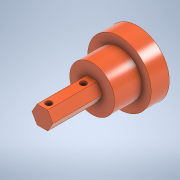
# Autodesk Inventor part: hexBushingForConnectorPiece
Saved by Autodesk Inventor 2022.2 (Build 262287000, 287)
## iProperties
Created: 2020-11-16
Part Number: hexBushingForConnectorPiece
Material: PC/ABS Plastic
Document SubType Name: Modeling
Designer: robst
Density: 0.357273 g/cm^3
Appearance: Smooth - Light Orange
Author: robst
Autodesk Inventor part; units mm, degrees
ref_plane "YZ Plane" through (0, 0, 0) normal (1, 0, 0) x (0, 1, 0)
ref_plane "XZ Plane" through (0, 0, 0) normal (0, 1, 0) x (-1, 0, 0)
ref_plane "XY Plane" through (0, 0, 0) normal (0, 0, 1) x (1, 0, 0)
sketch "Sketch1" plane through (0, 0, 0) normal (0, 0, 1) x (1, 0, 0)
  line L0 (7.3323, 0) -> (3.6662, -6.35)
  line L1 (3.6662, -6.35) -> (-3.6662, -6.35)
  line L2 (-3.6662, -6.35) -> (-7.3323, 0)
  line L3 (-7.3323, 0) -> (-3.6662, 6.35)
  line L4 (-3.6662, 6.35) -> (3.6662, 6.35)
  line L5 (3.6662, 6.35) -> (7.3323, 0)
  point P0 (0, 0)
  point P1 (0, 0)
  dimension "d0" = 12.7
  constraints: 12 end point, 1 coincident, 1 horizontal, 13 other
  measures "d0" distance between parallel lines of L1 L4
extrude "Extrusion1" add sketch "Sketch1" along normal mid plane 34.925
sketch "Sketch2" plane through (0, 0, -17.4625) normal (0, 0, -1) x (-1, 0, 0)
  circle A0 centre (0, 0) radius 15.748
  dimension "d3" = 31.496
  constraints: 1 centre point, 1 coincident
  measures "d3" diameter of A0
extrude "Extrusion2" add sketch "Sketch2" along normal blind 19.05
sketch "Sketch3" plane through (0, 0, -36.5125) normal (0, 0, -1) x (-1, 0, 0)
  circle A0 centre (0, 0) radius 22.225
  dimension "d6" = 44.45
  constraints: 1 centre point, 1 coincident
  measures "d6" diameter of A0
extrude "Extrusion3" add sketch "Sketch3" along normal blind 12.7
sketch "Sketch4" plane through (0, 0, -49.2125) normal (0, 0, -1) x (-1, 0, 0)
  circle A0 centre (0, 0) radius 16.51 construction
  line L0 (-13.6277, 3.4249) -> (-13.7163, 2.7889)
  line L1 (-13.7163, 2.7889) -> (-15.8691, 3.0889)
  spline S0 degree 2 poles (-15.8691, 3.0889) (-16.1301, 3.1253) (-16.5854, 3.1389) (-16.7302, 3.0842) knots 0 0 0 1 2 2 2
  spline S1 degree 2 poles (-16.7302, 3.0842) (-16.8837, 3.0267) (-17.061, 2.7687) (-17.0939, 2.5323) knots 0 0 0 1 2 2 2
  spline S2 degree 2 poles (-17.0939, 2.5323) (-17.1269, 2.2958) (-16.944, 1.759) (-16.7737, 1.4901) knots 0 0 0 1 2 2 2
  line L2 (-16.7737, 1.4901) -> (-13.9522, 1.0968)
  line L3 (-13.9522, 1.0968) -> (-14.0408, 0.4607)
  line L4 (-14.0408, 0.4607) -> (-19.2964, 1.1933)
  line L5 (-19.2964, 1.1933) -> (-19.2078, 1.8293)
  line L6 (-19.2078, 1.8293) -> (-17.3078, 1.5645)
  spline S3 degree 2 poles (-17.3078, 1.5645) (-17.5249, 1.8857) (-17.7172, 2.4737) (-17.6741, 2.7835) knots 0 0 0 1 2 2 2
  spline S4 degree 2 poles (-17.6741, 2.7835) (-17.5968, 3.338) (-16.7753, 3.8636) (-16.0781, 3.7665) knots 0 0 0 1 2 2 2
  line L7 (-16.0781, 3.7665) -> (-13.6277, 3.4249)
  spline S5 degree 2 poles (-12.6332, 5.765) (-12.9956, 4.9261) (-14.335, 4.4105) (-15.2042, 4.786) knots 0 0 0 1 2 2 2
  spline S6 degree 2 poles (-15.2042, 4.786) (-16.0582, 5.155) (-16.6841, 6.4882) (-16.3723, 7.21) knots 0 0 0 1 2 2 2
  spline S7 degree 2 poles (-16.3723, 7.21) (-16.2318, 7.535) (-15.8257, 7.956) (-15.5455, 8.0547) knots 0 0 0 1 2 2 2
  spline S8 degree 2 poles (-15.5455, 8.0547) (-15.2635, 8.1571) (-14.5988, 8.1076) (-14.1793, 7.9264) knots 0 0 0 1 2 2 2
  line L8 (-14.1793, 7.9264) -> (-13.8581, 7.7876)
  line L9 (-13.8581, 7.7876) -> (-14.9046, 5.3652)
  spline S9 degree 2 poles (-14.9046, 5.3652) (-14.2962, 5.1023) (-13.3855, 5.4353) (-13.1504, 5.9795) knots 0 0 0 1 2 2 2
  spline S10 degree 2 poles (-13.1504, 5.9795) (-13.0671, 6.1723) (-12.9924, 6.5839) (-12.9951, 6.7645) knots 0 0 0 1 2 2 2
  spline S11 degree 2 poles (-12.9951, 6.7645) (-13.0021, 6.9559) (-13.0397, 7.2322) (-13.0691, 7.3301) knots 0 0 0 1 2 2 2
  line L10 (-13.0691, 7.3301) -> (-13.0545, 7.3641)
  line L11 (-13.0545, 7.3641) -> (-12.412, 7.0866)
  spline S12 degree 2 poles (-12.412, 7.0866) (-12.4145, 6.9666) (-12.4275, 6.6045) (-12.4457, 6.4688) knots 0 0 0 1 2 2 2
  spline S13 degree 2 poles (-12.4457, 6.4688) (-12.47, 6.2776) (-12.5417, 5.9767) (-12.6332, 5.765) knots 0 0 0 1 2 2 2
  spline S14 degree 2 poles (-14.556, 7.4074) (-14.7973, 7.5027) (-15.1874, 7.5547) (-15.3454, 7.5108) knots 0 0 0 1 2 2 2
  spline S15 degree 2 poles (-15.3454, 7.5108) (-15.5218, 7.4659) (-15.8004, 7.2051) (-15.9032, 6.967) knots 0 0 0 1 2 2 2
  spline S16 degree 2 poles (-15.9032, 6.967) (-16.0045, 6.7327) (-16.0067, 6.3435) (-15.9294, 6.1487) knots 0 0 0 1 2 2 2
  spline S17 degree 2 poles (-15.9294, 6.1487) (-15.8467, 5.956) (-15.5692, 5.6747) (-15.3543, 5.5595) knots 0 0 0 1 2 2 2
  line L12 (-15.3543, 5.5595) -> (-14.556, 7.4074)
  line L13 (-9.9787, 9.9228) -> (-10.4619, 9.3025)
  line L14 (-10.4619, 9.3025) -> (-12.1613, 9.4521)
  line L15 (-12.1613, 9.4521) -> (-11.6155, 7.8216)
  line L16 (-11.6155, 7.8216) -> (-12.0633, 7.2467)
  line L17 (-12.0633, 7.2467) -> (-12.7419, 9.4504)
  line L18 (-12.7419, 9.4504) -> (-15.063, 9.599)
  line L19 (-15.063, 9.599) -> (-14.5799, 10.2193)
  line L20 (-14.5799, 10.2193) -> (-12.8927, 10.0741)
  line L21 (-12.8927, 10.0741) -> (-13.4339, 11.6905)
  line L22 (-13.4339, 11.6905) -> (-12.9861, 12.2654)
  line L23 (-12.9861, 12.2654) -> (-12.3089, 10.0733)
  line L24 (-12.3089, 10.0733) -> (-9.9787, 9.9228)
  spline S18 degree 2 poles (-7.7436, 13.5957) (-7.5175, 13.2918) (-7.4023, 12.6541) (-7.4808, 12.3596) knots 0 0 0 1 2 2 2
  spline S19 degree 2 poles (-7.4808, 12.3596) (-7.5794, 12.0093) (-7.9915, 11.4666) (-8.4077, 11.157) knots 0 0 0 1 2 2 2
  line L25 (-8.4077, 11.157) -> (-9.5769, 10.2872)
  line L26 (-9.5769, 10.2872) -> (-12.609, 14.3631)
  line L27 (-12.609, 14.3631) -> (-11.529, 15.1666)
  spline S20 degree 2 poles (-11.529, 15.1666) (-11.093, 15.4909) (-10.6152, 15.7591) (-10.336, 15.7975) knots 0 0 0 1 2 2 2
  spline S21 degree 2 poles (-10.336, 15.7975) (-10.0287, 15.8465) (-9.5446, 15.6166) (-9.3529, 15.359) knots 0 0 0 1 2 2 2
  spline S22 degree 2 poles (-9.3529, 15.359) (-9.1392, 15.0716) (-9.104, 14.3897) (-9.2757, 14.0619) knots 0 0 0 1 2 2 2
  line L28 (-9.2757, 14.0619) -> (-9.2609, 14.0421)
  spline S23 degree 2 poles (-9.2609, 14.0421) (-8.8239, 14.2133) (-8.0335, 13.9854) (-7.7436, 13.5957) knots 0 0 0 1 2 2 2
  spline S24 degree 2 poles (-8.2912, 13.1524) (-8.4632, 13.3836) (-8.8165, 13.5826) (-9.0933, 13.5408) knots 0 0 0 1 2 2 2
  spline S25 degree 2 poles (-9.0933, 13.5408) (-9.2712, 13.5111) (-9.6046, 13.3246) (-9.8853, 13.1158) knots 0 0 0 1 2 2 2
  line L29 (-9.8853, 13.1158) -> (-10.4997, 12.6587)
  line L30 (-10.4997, 12.6587) -> (-9.3792, 11.1526)
  line L31 (-9.3792, 11.1526) -> (-8.9399, 11.4794)
  spline S26 degree 2 poles (-8.9399, 11.4794) (-8.5832, 11.7448) (-8.2228, 12.1155) (-8.1429, 12.3391) knots 0 0 0 1 2 2 2
  spline S27 degree 2 poles (-8.1429, 12.3391) (-8.072, 12.5612) (-8.1315, 12.9377) (-8.2912, 13.1524) knots 0 0 0 1 2 2 2
  spline S28 degree 2 poles (-9.8612, 14.8628) (-9.9693, 15.0081) (-10.2306, 15.1524) (-10.3863, 15.1341) knots 0 0 0 1 2 2 2
  spline S29 degree 2 poles (-10.3863, 15.1341) (-10.5725, 15.1085) (-10.9174, 14.9032) (-11.2048, 14.6894) knots 0 0 0 1 2 2 2
  line L32 (-11.2048, 14.6894) -> (-11.7234, 14.3036)
  line L33 (-11.7234, 14.3036) -> (-10.8363, 13.1113)
  line L34 (-10.8363, 13.1113) -> (-10.222, 13.5683)
  spline S30 degree 2 poles (-10.222, 13.5683) (-9.9676, 13.7575) (-9.7658, 13.9897) (-9.6985, 14.1681) knots 0 0 0 1 2 2 2
  spline S31 degree 2 poles (-9.6985, 14.1681) (-9.6319, 14.3407) (-9.7187, 14.6712) (-9.8612, 14.8628) knots 0 0 0 1 2 2 2
  line L35 (-3.4638, 13.6147) -> (-4.066, 13.3916)
  line L36 (-4.066, 13.3916) -> (-4.2118, 13.7853)
  spline S32 degree 2 poles (-4.2118, 13.7853) (-4.3997, 13.4391) (-4.8047, 13.0037) (-5.1135, 12.8893) knots 0 0 0 1 2 2 2
  spline S33 degree 2 poles (-5.1135, 12.8893) (-5.3451, 12.8035) (-5.8154, 12.8049) (-6.0274, 12.9151) knots 0 0 0 1 2 2 2
  spline S34 degree 2 poles (-6.0274, 12.9151) (-6.2433, 13.0239) (-6.6006, 13.4666) (-6.735, 13.8295) knots 0 0 0 1 2 2 2
  line L37 (-6.735, 13.8295) -> (-7.5946, 16.1495)
  line L38 (-7.5946, 16.1495) -> (-6.9924, 16.3726)
  line L39 (-6.9924, 16.3726) -> (-6.2372, 14.3344)
  spline S35 degree 2 poles (-6.2372, 14.3344) (-6.1314, 14.0488) (-5.9502, 13.69) (-5.8253, 13.5782) knots 0 0 0 1 2 2 2
  spline S36 degree 2 poles (-5.8253, 13.5782) (-5.7005, 13.4665) (-5.4024, 13.432) (-5.1669, 13.5193) knots 0 0 0 1 2 2 2
  spline S37 degree 2 poles (-5.1669, 13.5193) (-4.9469, 13.6008) (-4.5419, 14.0362) (-4.4006, 14.2949) knots 0 0 0 1 2 2 2
  line L40 (-4.4006, 14.2949) -> (-5.3903, 16.9662)
  line L41 (-5.3903, 16.9662) -> (-4.7881, 17.1893)
  line L42 (-4.7881, 17.1893) -> (-3.4638, 13.6147)
  spline S38 degree 2 poles (-1.5215, 13.7959) (-1.9023, 13.7557) (-2.583, 13.8908) (-2.8121, 13.9825) knots 0 0 0 1 2 2 2
  line L43 (-2.8121, 13.9825) -> (-2.8878, 14.6989)
  line L44 (-2.8878, 14.6989) -> (-2.855, 14.7024)
  spline S39 degree 2 poles (-2.855, 14.7024) (-2.7662, 14.6455) (-2.5287, 14.5133) (-2.3354, 14.4468) knots 0 0 0 1 2 2 2
  spline S40 degree 2 poles (-2.3354, 14.4468) (-2.1676, 14.3859) (-1.7624, 14.3128) (-1.5536, 14.3348) knots 0 0 0 1 2 2 2
  spline S41 degree 2 poles (-1.5536, 14.3348) (-1.4022, 14.3508) (-1.0615, 14.4572) (-0.9857, 14.5231) knots 0 0 0 1 2 2 2
  spline S42 degree 2 poles (-0.9857, 14.5231) (-0.8752, 14.6135) (-0.7874, 14.8008) (-0.8064, 14.9809) knots 0 0 0 1 2 2 2
  spline S43 degree 2 poles (-0.8064, 14.9809) (-0.8302, 15.2061) (-1.1005, 15.4135) (-1.4239, 15.4579) knots 0 0 0 1 2 2 2
  spline S44 degree 2 poles (-1.4239, 15.4579) (-1.5498, 15.4736) (-1.9514, 15.514) (-2.124, 15.5413) knots 0 0 0 1 2 2 2
  spline S45 degree 2 poles (-2.124, 15.5413) (-2.5714, 15.6224) (-3.0198, 16.1049) (-3.0591, 16.4774) knots 0 0 0 1 2 2 2
  spline S46 degree 2 poles (-3.0591, 16.4774) (-3.1136, 16.9932) (-2.4078, 17.7177) (-1.7691, 17.7852) knots 0 0 0 1 2 2 2
  spline S47 degree 2 poles (-1.7691, 17.7852) (-1.4539, 17.8185) (-0.7988, 17.7304) (-0.5693, 17.6346) knots 0 0 0 1 2 2 2
  line L45 (-0.5693, 17.6346) -> (-0.497, 16.9509)
  line L46 (-0.497, 16.9509) -> (-0.5298, 16.9474)
  spline S48 degree 2 poles (-0.5298, 16.9474) (-0.7962, 17.118) (-1.4177, 17.28) (-1.7247, 17.2476) knots 0 0 0 1 2 2 2
  spline S49 degree 2 poles (-1.7247, 17.2476) (-2.04, 17.2143) (-2.4458, 16.9023) (-2.4177, 16.6362) knots 0 0 0 1 2 2 2
  spline S50 degree 2 poles (-2.4177, 16.6362) (-2.3922, 16.3947) (-2.1096, 16.1886) (-1.8153, 16.1452) knots 0 0 0 1 2 2 2
  spline S51 degree 2 poles (-1.8153, 16.1452) (-1.6722, 16.123) (-1.3123, 16.0865) (-1.1151, 16.0618) knots 0 0 0 1 2 2 2
  spline S52 degree 2 poles (-1.1151, 16.0618) (-0.6863, 15.9995) (-0.2091, 15.5573) (-0.1645, 15.1356) knots 0 0 0 1 2 2 2
  spline S53 degree 2 poles (-0.1645, 15.1356) (-0.1386, 14.89) (-0.2852, 14.4357) (-0.4566, 14.2562) knots 0 0 0 1 2 2 2
  spline S54 degree 2 poles (-0.4566, 14.2562) (-0.6395, 14.0671) (-1.1326, 13.837) (-1.5215, 13.7959) knots 0 0 0 1 2 2 2
  line L47 (3.5043, 13.6075) -> (2.8688, 13.6998)
  line L48 (2.8688, 13.6998) -> (3.1814, 15.8509)
  spline S55 degree 2 poles (3.1814, 15.8509) (3.2193, 16.1116) (3.2355, 16.5668) (3.1817, 16.7119) knots 0 0 0 1 2 2 2
  spline S56 degree 2 poles (3.1817, 16.7119) (3.125, 16.8658) (2.8681, 17.0445) (2.6319, 17.0789) knots 0 0 0 1 2 2 2
  spline S57 degree 2 poles (2.6319, 17.0789) (2.3956, 17.1132) (1.8578, 16.9334) (1.5878, 16.7647) knots 0 0 0 1 2 2 2
  line L49 (1.5878, 16.7647) -> (1.1781, 13.9455)
  line L50 (1.1781, 13.9455) -> (0.5426, 14.0379)
  line L51 (0.5426, 14.0379) -> (1.3057, 19.2892)
  line L52 (1.3057, 19.2892) -> (1.9413, 19.1968)
  line L53 (1.9413, 19.1968) -> (1.6654, 17.2984)
  spline S58 degree 2 poles (1.6654, 17.2984) (1.9878, 17.5136) (2.5769, 17.7025) (2.8865, 17.6575) knots 0 0 0 1 2 2 2
  spline S59 degree 2 poles (2.8865, 17.6575) (3.4406, 17.577) (3.9614, 16.7525) (3.8601, 16.0559) knots 0 0 0 1 2 2 2
  line L54 (3.8601, 16.0559) -> (3.5043, 13.6075)
  line L55 (4.9605, 13.0636) -> (4.355, 13.2777)
  line L56 (4.355, 13.2777) -> (5.626, 16.8717)
  line L57 (5.626, 16.8717) -> (6.2315, 16.6575)
  line L58 (6.2315, 16.6575) -> (4.9605, 13.0636)
  line L59 (6.4855, 17.2401) -> (5.7986, 17.4831)
  line L60 (5.7986, 17.4831) -> (6.0209, 18.1118)
  line L61 (6.0209, 18.1118) -> (6.7079, 17.8689)
  line L62 (6.7079, 17.8689) -> (6.4855, 17.2401)
  line L63 (8.428, 11.2433) -> (7.8757, 11.571)
  line L64 (7.8757, 11.571) -> (8.9849, 13.4403)
  spline S60 degree 2 poles (8.9849, 13.4403) (9.1193, 13.6669) (9.3079, 14.0816) (9.3135, 14.2362) knots 0 0 0 1 2 2 2
  spline S61 degree 2 poles (9.3135, 14.2362) (9.3198, 14.4001) (9.1504, 14.6633) (8.9451, 14.7851) knots 0 0 0 1 2 2 2
  spline S62 degree 2 poles (8.9451, 14.7851) (8.7398, 14.907) (8.174, 14.9458) (7.8601, 14.8928) knots 0 0 0 1 2 2 2
  line L65 (7.8601, 14.8928) -> (6.4064, 12.4428)
  line L66 (6.4064, 12.4428) -> (5.8542, 12.7705)
  line L67 (5.8542, 12.7705) -> (7.7994, 16.0489)
  line L68 (7.7994, 16.0489) -> (8.3517, 15.7212)
  line L69 (8.3517, 15.7212) -> (8.1353, 15.3565)
  spline S63 degree 2 poles (8.1353, 15.3565) (8.5155, 15.4325) (9.1321, 15.3826) (9.4012, 15.223) knots 0 0 0 1 2 2 2
  spline S64 degree 2 poles (9.4012, 15.223) (9.8826, 14.9373) (10.0497, 13.9765) (9.6905, 13.3711) knots 0 0 0 1 2 2 2
  line L70 (9.6905, 13.3711) -> (8.428, 11.2433)
  spline S65 degree 2 poles (8.7739, 10.1635) (8.7983, 10.0959) (8.9055, 9.8514) (8.9892, 9.7095) knots 0 0 0 1 2 2 2
  spline S66 degree 2 poles (8.9892, 9.7095) (9.0782, 9.5499) (9.2463, 9.2951) (9.3682, 9.1668) knots 0 0 0 1 2 2 2
  spline S67 degree 2 poles (9.3682, 9.1668) (9.5723, 8.9518) (9.9692, 8.761) (10.1501, 8.7737) knots 0 0 0 1 2 2 2
  spline S68 degree 2 poles (10.1501, 8.7737) (10.3281, 8.7895) (10.6533, 8.9791) (10.8235, 9.1406) knots 0 0 0 1 2 2 2
  line L71 (10.8235, 9.1406) -> (11.0653, 9.3702)
  spline S69 degree 2 poles (11.0653, 9.3702) (10.7226, 9.4024) (10.2243, 9.6163) (9.9664, 9.8879) knots 0 0 0 1 2 2 2
  spline S70 degree 2 poles (9.9664, 9.8879) (9.5186, 10.3597) (9.6901, 11.584) (10.3499, 12.2104) knots 0 0 0 1 2 2 2
  spline S71 degree 2 poles (10.3499, 12.2104) (10.6932, 12.5364) (11.4089, 12.8469) (11.75, 12.8642) knots 0 0 0 1 2 2 2
  spline S72 degree 2 poles (11.75, 12.8642) (12.0736, 12.8762) (12.673, 12.6335) (12.8884, 12.4066) knots 0 0 0 1 2 2 2
  spline S73 degree 2 poles (12.8884, 12.4066) (13.0925, 12.1917) (13.2886, 11.7818) (13.3462, 11.5357) knots 0 0 0 1 2 2 2
  line L72 (13.3462, 11.5357) -> (13.4882, 11.6194)
  line L73 (13.4882, 11.6194) -> (13.9048, 11.1806)
  line L74 (13.9048, 11.1806) -> (11.4568, 8.8563)
  spline S74 degree 2 poles (11.4568, 8.8563) (10.7522, 8.1874) (9.5143, 8.1758) (8.9162, 8.8058) knots 0 0 0 1 2 2 2
  spline S75 degree 2 poles (8.9162, 8.8058) (8.7235, 9.0088) (8.3867, 9.4951) (8.2675, 9.7282) knots 0 0 0 1 2 2 2
  line L75 (8.2675, 9.7282) -> (8.7512, 10.1874)
  line L76 (8.7512, 10.1874) -> (8.7739, 10.1635)
  line L77 (11.4475, 9.733) -> (12.9671, 11.1758)
  spline S76 degree 2 poles (12.9671, 11.1758) (12.8863, 11.4283) (12.6802, 11.7889) (12.5413, 11.9352) knots 0 0 0 1 2 2 2
  spline S77 degree 2 poles (12.5413, 11.9352) (12.2068, 12.2875) (11.3018, 12.2003) (10.8152, 11.7383) knots 0 0 0 1 2 2 2
  spline S78 degree 2 poles (10.8152, 11.7383) (10.3554, 11.3018) (10.1667, 10.5379) (10.4955, 10.1916) knots 0 0 0 1 2 2 2
  spline S79 degree 2 poles (10.4955, 10.1916) (10.6684, 10.0095) (11.1745, 9.7634) (11.4475, 9.733) knots 0 0 0 1 2 2 2
  line L78 (17.0752, 7.1971) -> (15.958, 9.2793)
  line L79 (15.958, 9.2793) -> (14.6956, 8.602)
  line L80 (14.6956, 8.602) -> (15.7661, 6.6068)
  line L81 (15.7661, 6.6068) -> (15.2365, 6.3227)
  line L82 (15.2365, 6.3227) -> (14.166, 8.3178)
  line L83 (14.166, 8.3178) -> (12.0113, 7.1617)
  line L84 (12.0113, 7.1617) -> (11.6921, 7.7566)
  line L85 (11.6921, 7.7566) -> (16.1684, 10.1584)
  line L86 (16.1684, 10.1584) -> (17.6048, 7.4812)
  line L87 (17.6048, 7.4812) -> (17.0752, 7.1971)
  spline S80 degree 2 poles (15.8501, 1.9288) (14.9117, 1.7112) (13.6798, 2.3763) (13.5049, 3.1302) knots 0 0 0 1 2 2 2
  spline S81 degree 2 poles (13.5049, 3.1302) (13.3254, 3.9042) (14.1746, 5.0351) (15.0809, 5.2453) knots 0 0 0 1 2 2 2
  spline S82 degree 2 poles (15.0809, 5.2453) (16.0112, 5.4611) (17.2539, 4.7858) (17.427, 4.0399) knots 0 0 0 1 2 2 2
  spline S83 degree 2 poles (17.427, 4.0399) (17.6018, 3.286) (16.7845, 2.1456) (15.8501, 1.9288) knots 0 0 0 1 2 2 2
  spline S84 degree 2 poles (15.7003, 2.5745) (16.4222, 2.7419) (17.0021, 3.43) (16.8896, 3.9153) knots 0 0 0 1 2 2 2
  spline S85 degree 2 poles (16.8896, 3.9153) (16.777, 4.4005) (15.9525, 4.7671) (15.2306, 4.5997) knots 0 0 0 1 2 2 2
  spline S86 degree 2 poles (15.2306, 4.5997) (14.5288, 4.4369) (13.9298, 3.7401) (14.0423, 3.2549) knots 0 0 0 1 2 2 2
  spline S87 degree 2 poles (14.0423, 3.2549) (14.1539, 2.7736) (14.9865, 2.4089) (15.7003, 2.5745) knots 0 0 0 1 2 2 2
  line L88 (17.0983, -1.1737) -> (17.0982, -1.1408)
  spline S88 degree 2 poles (17.0982, -1.1408) (17.1185, -1.0666) (17.1263, -0.906) (17.1259, -0.7949) knots 0 0 0 1 2 2 2
  spline S89 degree 2 poles (17.1259, -0.7949) (17.1251, -0.5355) (16.8971, -0.0258) (16.6741, 0.2041) knots 0 0 0 1 2 2 2
  line L89 (16.6741, 0.2041) -> (13.9695, 0.1957)
  line L90 (13.9695, 0.1957) -> (13.9675, 0.8379)
  line L91 (13.9675, 0.8379) -> (17.7795, 0.8497)
  line L92 (17.7795, 0.8497) -> (17.7815, 0.2075)
  line L93 (17.7815, 0.2075) -> (17.2134, 0.2058)
  spline S90 degree 2 poles (17.2134, 0.2058) (17.5274, -0.1432) (17.7842, -0.6652) (17.785, -0.9122) knots 0 0 0 1 2 2 2
  spline S91 degree 2 poles (17.785, -0.9122) (17.7853, -1.011) (17.7774, -1.1098) (17.7652, -1.1716) knots 0 0 0 1 2 2 2
  line L94 (17.7652, -1.1716) -> (17.0983, -1.1737)
  spline S92 degree 2 poles (13.4014, -3.6335) (13.5168, -3.1532) (14.0363, -2.4185) (14.4317, -2.2002) knots 0 0 0 1 2 2 2
  spline S93 degree 2 poles (14.4317, -2.2002) (14.8231, -1.981) (15.8617, -1.8876) (16.4861, -2.0377) knots 0 0 0 1 2 2 2
  spline S94 degree 2 poles (16.4861, -2.0377) (17.1066, -2.1868) (17.9512, -2.7243) (18.2193, -3.1062) knots 0 0 0 1 2 2 2
  spline S95 degree 2 poles (18.2193, -3.1062) (18.4803, -3.4823) (18.6342, -4.3745) (18.514, -4.8749) knots 0 0 0 1 2 2 2
  spline S96 degree 2 poles (18.514, -4.8749) (18.4544, -5.123) (18.2775, -5.542) (18.1772, -5.7127) knots 0 0 0 1 2 2 2
  spline S97 degree 2 poles (18.1772, -5.7127) (18.0867, -5.8603) (17.8587, -6.1569) (17.7312, -6.2999) knots 0 0 0 1 2 2 2
  line L95 (17.7312, -6.2999) -> (16.9387, -6.1094)
  line L96 (16.9387, -6.1094) -> (16.9512, -6.0574)
  spline S98 degree 2 poles (16.9512, -6.0574) (17.0524, -5.9885) (17.342, -5.7702) (17.4972, -5.6001) knots 0 0 0 1 2 2 2
  spline S99 degree 2 poles (17.4972, -5.6001) (17.6465, -5.4369) (17.8853, -5.0244) (17.9546, -4.7362) knots 0 0 0 1 2 2 2
  spline S100 degree 2 poles (17.9546, -4.7362) (18.0306, -4.42) (17.906, -3.7931) (17.7088, -3.5213) knots 0 0 0 1 2 2 2
  spline S101 degree 2 poles (17.7088, -3.5213) (17.5067, -3.2525) (16.798, -2.8366) (16.3216, -2.7222) knots 0 0 0 1 2 2 2
  spline S102 degree 2 poles (16.3216, -2.7222) (15.8133, -2.6) (15.0221, -2.6681) (14.719, -2.8197) knots 0 0 0 1 2 2 2
  spline S103 degree 2 poles (14.719, -2.8197) (14.4248, -2.9691) (14.0429, -3.4659) (13.9679, -3.7781) knots 0 0 0 1 2 2 2
  spline S104 degree 2 poles (13.9679, -3.7781) (13.8996, -4.0623) (13.9233, -4.5803) (13.9821, -4.7934) knots 0 0 0 1 2 2 2
  spline S105 degree 2 poles (13.9821, -4.7934) (14.0429, -4.9985) (14.1946, -5.3187) (14.2524, -5.413) knots 0 0 0 1 2 2 2
  line L97 (14.2524, -5.413) -> (14.2408, -5.461)
  line L98 (14.2408, -5.461) -> (13.4563, -5.2725)
  spline S106 degree 2 poles (13.4563, -5.2725) (13.4197, -5.0901) (13.3489, -4.7682) (13.3339, -4.5487) knots 0 0 0 1 2 2 2
  spline S107 degree 2 poles (13.3339, -4.5487) (13.3138, -4.3152) (13.3302, -3.9297) (13.4014, -3.6335) knots 0 0 0 1 2 2 2
  spline S108 degree 2 poles (12.934, -9.3626) (12.0979, -8.8841) (11.6468, -7.5588) (12.0312, -6.8871) knots 0 0 0 1 2 2 2
  spline S109 degree 2 poles (12.0312, -6.8871) (12.4258, -6.1975) (13.8174, -5.9456) (14.6249, -6.4076) knots 0 0 0 1 2 2 2
  spline S110 degree 2 poles (14.6249, -6.4076) (15.4539, -6.882) (15.906, -8.2221) (15.5257, -8.8867) knots 0 0 0 1 2 2 2
  spline S111 degree 2 poles (15.5257, -8.8867) (15.1413, -9.5584) (13.7665, -9.839) (12.934, -9.3626) knots 0 0 0 1 2 2 2
  spline S112 degree 2 poles (13.2632, -8.7873) (13.9063, -9.1553) (14.7995, -9.0451) (15.0469, -8.6127) knots 0 0 0 1 2 2 2
  spline S113 degree 2 poles (15.0469, -8.6127) (15.2943, -8.1804) (14.9389, -7.3509) (14.2957, -6.9829) knots 0 0 0 1 2 2 2
  spline S114 degree 2 poles (14.2957, -6.9829) (13.6704, -6.6251) (12.7574, -6.7287) (12.51, -7.161) knots 0 0 0 1 2 2 2
  spline S115 degree 2 poles (12.51, -7.161) (12.2646, -7.5898) (12.6272, -8.4234) (13.2632, -8.7873) knots 0 0 0 1 2 2 2
  line L99 (8.7251, -11.0143) -> (9.1827, -10.5637)
  line L100 (9.1827, -10.5637) -> (10.7078, -12.1125)
  spline S116 degree 2 poles (10.7078, -12.1125) (10.8927, -12.3003) (11.2456, -12.5883) (11.3937, -12.6331) knots 0 0 0 1 2 2 2
  spline S117 degree 2 poles (11.3937, -12.6331) (11.5505, -12.6809) (11.8482, -12.5842) (12.0183, -12.4167) knots 0 0 0 1 2 2 2
  spline S118 degree 2 poles (12.0183, -12.4167) (12.1885, -12.2492) (12.3702, -11.712) (12.3988, -11.3949) knots 0 0 0 1 2 2 2
  line L101 (12.3988, -11.3949) -> (10.4001, -9.3651)
  line L102 (10.4001, -9.3651) -> (10.8577, -8.9145)
  line L103 (10.8577, -8.9145) -> (13.5323, -11.6308)
  line L104 (13.5323, -11.6308) -> (13.0747, -12.0813)
  line L105 (13.0747, -12.0813) -> (12.7772, -11.7792)
  spline S119 degree 2 poles (12.7772, -11.7792) (12.7538, -12.1662) (12.5485, -12.7497) (12.3255, -12.9692) knots 0 0 0 1 2 2 2
  spline S120 degree 2 poles (12.3255, -12.9692) (11.9266, -13.3621) (10.955, -13.2789) (10.4611, -12.7773) knots 0 0 0 1 2 2 2
  line L106 (10.4611, -12.7773) -> (8.7251, -11.0143)
  line L107 (5.3806, -12.9805) -> (5.944, -12.6722)
  line L108 (5.944, -12.6722) -> (6.9874, -14.579)
  spline S121 degree 2 poles (6.9874, -14.579) (7.1139, -14.8101) (7.3746, -15.1836) (7.5048, -15.2673) knots 0 0 0 1 2 2 2
  spline S122 degree 2 poles (7.5048, -15.2673) (7.6426, -15.3561) (7.9554, -15.3445) (8.1648, -15.2299) knots 0 0 0 1 2 2 2
  spline S123 degree 2 poles (8.1648, -15.2299) (8.3743, -15.1153) (8.696, -14.6483) (8.8102, -14.3511) knots 0 0 0 1 2 2 2
  line L109 (8.8102, -14.3511) -> (7.4427, -11.8521)
  line L110 (7.4427, -11.8521) -> (8.0061, -11.5438)
  line L111 (8.0061, -11.5438) -> (9.836, -14.8879)
  line L112 (9.836, -14.8879) -> (9.2727, -15.1962)
  line L113 (9.2727, -15.1962) -> (9.0691, -14.8242)
  spline S124 degree 2 poles (9.0691, -14.8242) (8.9408, -15.1901) (8.5837, -15.6952) (8.3092, -15.8454) knots 0 0 0 1 2 2 2
  spline S125 degree 2 poles (8.3092, -15.8454) (7.8181, -16.1142) (6.9062, -15.7684) (6.5683, -15.1509) knots 0 0 0 1 2 2 2
  line L114 (6.5683, -15.1509) -> (5.3806, -12.9805)
  spline S126 degree 2 poles (2.9092, -13.5782) (3.7988, -13.3687) (5.0115, -14.1361) (5.2287, -15.0577) knots 0 0 0 1 2 2 2
  spline S127 degree 2 poles (5.2287, -15.0577) (5.442, -15.9633) (4.7454, -17.2609) (3.98, -17.4412) knots 0 0 0 1 2 2 2
  spline S128 degree 2 poles (3.98, -17.4412) (3.6354, -17.5224) (3.0553, -17.4476) (2.8089, -17.2815) knots 0 0 0 1 2 2 2
  spline S129 degree 2 poles (2.8089, -17.2815) (2.5585, -17.1163) (2.2017, -16.5533) (2.0969, -16.1085) knots 0 0 0 1 2 2 2
  line L115 (2.0969, -16.1085) -> (2.0167, -15.7679)
  line L116 (2.0167, -15.7679) -> (4.5852, -15.1628)
  spline S130 degree 2 poles (4.5852, -15.1628) (4.4332, -14.5176) (3.6226, -13.9854) (3.0456, -14.1213) knots 0 0 0 1 2 2 2
  spline S131 degree 2 poles (3.0456, -14.1213) (2.8413, -14.1695) (2.4663, -14.3551) (2.323, -14.465) knots 0 0 0 1 2 2 2
  spline S132 degree 2 poles (2.323, -14.465) (2.1736, -14.5848) (1.9742, -14.7797) (1.9132, -14.8618) knots 0 0 0 1 2 2 2
  line L117 (1.9132, -14.8618) -> (1.8771, -14.8703)
  line L118 (1.8771, -14.8703) -> (1.7167, -14.1891)
  spline S133 degree 2 poles (1.7167, -14.1891) (1.8145, -14.1195) (2.1128, -13.9139) (2.2325, -13.8476) knots 0 0 0 1 2 2 2
  spline S134 degree 2 poles (2.2325, -13.8476) (2.4006, -13.7531) (2.6848, -13.6311) (2.9092, -13.5782) knots 0 0 0 1 2 2 2
  spline S135 degree 2 poles (2.7381, -16.1012) (2.8056, -16.3518) (2.9966, -16.6959) (3.1261, -16.7965) knots 0 0 0 1 2 2 2
  spline S136 degree 2 poles (3.1261, -16.7965) (3.2673, -16.9112) (3.6428, -16.9793) (3.8953, -16.9198) knots 0 0 0 1 2 2 2
  spline S137 degree 2 poles (3.8953, -16.9198) (4.1437, -16.8613) (4.4574, -16.6309) (4.5676, -16.4526) knots 0 0 0 1 2 2 2
  spline S138 degree 2 poles (4.5676, -16.4526) (4.673, -16.2713) (4.7332, -15.8807) (4.6975, -15.6396) knots 0 0 0 1 2 2 2
  line L119 (4.6975, -15.6396) -> (2.7381, -16.1012)
  spline S139 degree 2 poles (-0.5671, -13.8769) (-0.1719, -13.8825) (0.4791, -14.1347) (0.7102, -14.3851) knots 0 0 0 1 2 2 2
  spline S140 degree 2 poles (0.7102, -14.3851) (0.9414, -14.6313) (1.19, -15.3842) (1.1828, -15.8863) knots 0 0 0 1 2 2 2
  spline S141 degree 2 poles (1.1828, -15.8863) (1.1756, -16.3885) (0.8975, -17.1174) (0.6676, -17.3611) knots 0 0 0 1 2 2 2
  spline S142 degree 2 poles (0.6676, -17.3611) (0.4376, -17.609) (-0.2372, -17.8669) (-0.6241, -17.8614) knots 0 0 0 1 2 2 2
  spline S143 degree 2 poles (-0.6241, -17.8614) (-0.9369, -17.8569) (-1.5189, -17.6716) (-1.7436, -17.5531) knots 0 0 0 1 2 2 2
  line L120 (-1.7436, -17.5531) -> (-1.7333, -16.8327)
  line L121 (-1.7333, -16.8327) -> (-1.6963, -16.8333)
  spline S144 degree 2 poles (-1.6963, -16.8333) (-1.6271, -16.8919) (-1.4152, -17.0431) (-1.264, -17.1235) knots 0 0 0 1 2 2 2
  spline S145 degree 2 poles (-1.264, -17.1235) (-1.1291, -17.1913) (-0.7684, -17.2994) (-0.6037, -17.3018) knots 0 0 0 1 2 2 2
  spline S146 degree 2 poles (-0.6037, -17.3018) (-0.1057, -17.3089) (0.5102, -16.5643) (0.5201, -15.8769) knots 0 0 0 1 2 2 2
  spline S147 degree 2 poles (0.5201, -15.8769) (0.5297, -15.2059) (-0.0441, -14.4443) (-0.5627, -14.4368) knots 0 0 0 1 2 2 2
  spline S148 degree 2 poles (-0.5627, -14.4368) (-0.8756, -14.4324) (-1.4473, -14.6836) (-1.6684, -14.8821) knots 0 0 0 1 2 2 2
  line L122 (-1.6684, -14.8821) -> (-1.7054, -14.8816)
  line L123 (-1.7054, -14.8816) -> (-1.6951, -14.1613)
  spline S149 degree 2 poles (-1.6951, -14.1613) (-1.5998, -14.1173) (-1.3098, -13.9939) (-1.1942, -13.9667) knots 0 0 0 1 2 2 2
  spline S150 degree 2 poles (-1.1942, -13.9667) (-1.0288, -13.9197) (-0.7688, -13.874) (-0.5671, -13.8769) knots 0 0 0 1 2 2 2
  spline S151 degree 2 poles (-3.3715, -13.4881) (-2.8605, -13.5985) (-2.4111, -14.3062) (-2.5475, -14.938) knots 0 0 0 1 2 2 2
  line L124 (-2.5475, -14.938) -> (-2.9932, -17.0023)
  line L125 (-2.9932, -17.0023) -> (-2.5707, -17.0935)
  line L126 (-2.5707, -17.0935) -> (-2.6828, -17.6126)
  line L127 (-2.6828, -17.6126) -> (-3.1053, -17.5214)
  line L128 (-3.1053, -17.5214) -> (-3.3364, -18.5917)
  line L129 (-3.3364, -18.5917) -> (-3.9642, -18.4562)
  line L130 (-3.9642, -18.4562) -> (-3.733, -17.3858)
  line L131 (-3.733, -17.3858) -> (-4.8879, -17.1364)
  line L132 (-4.8879, -17.1364) -> (-4.7758, -16.6173)
  line L133 (-4.7758, -16.6173) -> (-3.621, -16.8667)
  line L134 (-3.621, -16.8667) -> (-3.2378, -15.0922)
  spline S152 degree 2 poles (-3.2378, -15.0922) (-3.177, -14.8105) (-3.1302, -14.4963) (-3.1699, -14.3487) knots 0 0 0 1 2 2 2
  spline S153 degree 2 poles (-3.1699, -14.3487) (-3.201, -14.2199) (-3.4294, -14.0484) (-3.6466, -14.0015) knots 0 0 0 1 2 2 2
  spline S154 degree 2 poles (-3.6466, -14.0015) (-3.7996, -13.9685) (-4.1052, -13.9994) (-4.1757, -14.0136) knots 0 0 0 1 2 2 2
  line L135 (-4.1757, -14.0136) -> (-4.2119, -14.0058)
  line L136 (-4.2119, -14.0058) -> (-4.0903, -13.4424)
  spline S155 degree 2 poles (-4.0903, -13.4424) (-3.9028, -13.4324) (-3.5285, -13.4543) (-3.3715, -13.4881) knots 0 0 0 1 2 2 2
  spline S156 degree 2 poles (-8.1797, -13.7127) (-7.7773, -12.8375) (-6.4971, -12.2707) (-5.794, -12.5941) knots 0 0 0 1 2 2 2
  spline S157 degree 2 poles (-5.794, -12.5941) (-5.0721, -12.9261) (-4.6979, -14.2899) (-5.0866, -15.1351) knots 0 0 0 1 2 2 2
  spline S158 degree 2 poles (-5.0866, -15.1351) (-5.4857, -16.0028) (-6.7805, -16.5719) (-7.4761, -16.252) knots 0 0 0 1 2 2 2
  spline S159 degree 2 poles (-7.4761, -16.252) (-8.1793, -15.9286) (-8.5805, -14.5841) (-8.1797, -13.7127) knots 0 0 0 1 2 2 2
  spline S160 degree 2 poles (-7.5776, -13.9896) (-7.8872, -14.6628) (-7.6982, -15.5427) (-7.2457, -15.7508) knots 0 0 0 1 2 2 2
  spline S161 degree 2 poles (-7.2457, -15.7508) (-6.7931, -15.9589) (-5.9984, -15.5314) (-5.6888, -14.8582) knots 0 0 0 1 2 2 2
  spline S162 degree 2 poles (-5.6888, -14.8582) (-5.3878, -14.2037) (-5.5719, -13.3034) (-6.0245, -13.0953) knots 0 0 0 1 2 2 2
  spline S163 degree 2 poles (-6.0245, -13.0953) (-6.4733, -12.8889) (-7.2714, -13.3239) (-7.5776, -13.9896) knots 0 0 0 1 2 2 2
  line L137 (-11.397, -12.7999) -> (-11.3709, -12.82)
  spline S164 degree 2 poles (-11.3709, -12.82) (-11.3247, -12.8815) (-11.2025, -12.9859) (-11.1144, -13.0537) knots 0 0 0 1 2 2 2
  spline S165 degree 2 poles (-11.1144, -13.0537) (-10.9088, -13.2119) (-10.3662, -13.3437) (-10.0479, -13.3081) knots 0 0 0 1 2 2 2
  line L138 (-10.0479, -13.3081) -> (-8.3986, -11.1646)
  line L139 (-8.3986, -11.1646) -> (-7.8896, -11.5562)
  line L140 (-7.8896, -11.5562) -> (-10.2143, -14.5774)
  line L141 (-10.2143, -14.5774) -> (-10.7233, -14.1858)
  line L142 (-10.7233, -14.1858) -> (-10.3768, -13.7355)
  spline S166 degree 2 poles (-10.3768, -13.7355) (-10.8449, -13.7701) (-11.4149, -13.6536) (-11.6107, -13.5029) knots 0 0 0 1 2 2 2
  spline S167 degree 2 poles (-11.6107, -13.5029) (-11.689, -13.4427) (-11.7623, -13.3759) (-11.8037, -13.3285) knots 0 0 0 1 2 2 2
  line L143 (-11.8037, -13.3285) -> (-11.397, -12.7999)
  spline S168 degree 2 poles (-8.0479, 4.6791) (-7.7366, 4.5717) (-7.2527, 4.1566) (-7.1266, 3.891) knots 0 0 0 1 2 2 2
  spline S169 degree 2 poles (-7.1266, 3.891) (-6.9673, 3.5574) (-6.9466, 2.7968) (-7.1238, 2.2831) knots 0 0 0 1 2 2 2
  line L144 (-7.1238, 2.2831) -> (-7.3104, 1.7422)
  line L145 (-7.3104, 1.7422) -> (-5.5202, 1.1247)
  line L146 (-5.5202, 1.1247) -> (-5.7404, 0.4865)
  line L147 (-5.7404, 0.4865) -> (-10.5427, 2.143)
  line L148 (-10.5427, 2.143) -> (-10.1265, 3.3494)
  spline S170 degree 2 poles (-10.1265, 3.3494) (-9.9789, 3.7775) (-9.632, 4.3285) (-9.3933, 4.5031) knots 0 0 0 1 2 2 2
  spline S171 degree 2 poles (-9.3933, 4.5031) (-9.1177, 4.7085) (-8.4487, 4.8174) (-8.0479, 4.6791) knots 0 0 0 1 2 2 2
  spline S172 degree 2 poles (-8.258, 4.0069) (-8.507, 4.0929) (-8.9319, 4.0478) (-9.1091, 3.913) knots 0 0 0 1 2 2 2
  spline S173 degree 2 poles (-9.1091, 3.913) (-9.2626, 3.7961) (-9.484, 3.4195) (-9.5873, 3.1199) knots 0 0 0 1 2 2 2
  line L149 (-9.5873, 3.1199) -> (-9.7699, 2.5906)
  line L150 (-9.7699, 2.5906) -> (-7.8552, 1.9301)
  line L151 (-7.8552, 1.9301) -> (-7.7049, 2.366)
  spline S174 degree 2 poles (-7.7049, 2.366) (-7.5706, 2.7552) (-7.53, 3.2768) (-7.6398, 3.4889) knots 0 0 0 1 2 2 2
  spline S175 degree 2 poles (-7.6398, 3.4889) (-7.7341, 3.6825) (-8.0284, 3.9277) (-8.258, 4.0069) knots 0 0 0 1 2 2 2
  line L152 (-3.6339, 4.2535) -> (-4.0974, 3.809)
  line L153 (-4.0974, 3.809) -> (-6.7359, 6.5605)
  line L154 (-6.7359, 6.5605) -> (-6.2723, 7.005)
  line L155 (-6.2723, 7.005) -> (-3.6339, 4.2535)
  line L156 (-6.6784, 7.4939) -> (-7.2044, 6.9896)
  line L157 (-7.2044, 6.9896) -> (-7.666, 7.4709)
  line L158 (-7.666, 7.4709) -> (-7.14, 7.9752)
  line L159 (-7.14, 7.9752) -> (-6.6784, 7.4939)
  spline S176 degree 2 poles (-1.3794, 5.3304) (-2.2513, 5.0564) (-3.5169, 5.7332) (-3.8007, 6.6365) knots 0 0 0 1 2 2 2
  spline S177 degree 2 poles (-3.8007, 6.6365) (-4.0796, 7.5241) (-3.4796, 8.8691) (-2.7294, 9.1048) knots 0 0 0 1 2 2 2
  spline S178 degree 2 poles (-2.7294, 9.1048) (-2.3917, 9.211) (-1.8076, 9.1787) (-1.5498, 9.031) knots 0 0 0 1 2 2 2
  spline S179 degree 2 poles (-1.5498, 9.031) (-1.288, 8.8846) (-0.8911, 8.3491) (-0.7541, 7.9132) knots 0 0 0 1 2 2 2
  line L160 (-0.7541, 7.9132) -> (-0.6492, 7.5794)
  line L161 (-0.6492, 7.5794) -> (-3.1666, 6.7883)
  spline S180 degree 2 poles (-3.1666, 6.7883) (-2.9679, 6.156) (-2.1206, 5.6843) (-1.5551, 5.862) knots 0 0 0 1 2 2 2
  spline S181 degree 2 poles (-1.5551, 5.862) (-1.3548, 5.925) (-0.9944, 6.1375) (-0.8595, 6.2576) knots 0 0 0 1 2 2 2
  spline S182 degree 2 poles (-0.8595, 6.2576) (-0.7192, 6.3879) (-0.5346, 6.597) (-0.4798, 6.6833) knots 0 0 0 1 2 2 2
  line L162 (-0.4798, 6.6833) -> (-0.4444, 6.6944)
  line L163 (-0.4444, 6.6944) -> (-0.2346, 6.0267)
  spline S183 degree 2 poles (-0.2346, 6.0267) (-0.3271, 5.9502) (-0.6096, 5.7233) (-0.7242, 5.6485) knots 0 0 0 1 2 2 2
  spline S184 degree 2 poles (-0.7242, 5.6485) (-0.8849, 5.5419) (-1.1595, 5.3995) (-1.3794, 5.3304) knots 0 0 0 1 2 2 2
  spline S185 degree 2 poles (-1.393, 7.8591) (-1.4786, 8.1041) (-1.6942, 8.4333) (-1.8307, 8.5242) knots 0 0 0 1 2 2 2
  spline S186 degree 2 poles (-1.8307, 8.5242) (-1.9799, 8.6283) (-2.3594, 8.6688) (-2.6068, 8.591) knots 0 0 0 1 2 2 2
  spline S187 degree 2 poles (-2.6068, 8.591) (-2.8503, 8.5145) (-3.1463, 8.2618) (-3.2433, 8.076) knots 0 0 0 1 2 2 2
  spline S188 degree 2 poles (-3.2433, 8.076) (-3.3351, 7.8875) (-3.3666, 7.4935) (-3.3135, 7.2556) knots 0 0 0 1 2 2 2
  line L164 (-3.3135, 7.2556) -> (-1.393, 7.8591)
  spline S189 degree 2 poles (1.9482, 5.1553) (1.57, 5.2699) (1.014, 5.6923) (0.8612, 5.9968) knots 0 0 0 1 2 2 2
  spline S190 degree 2 poles (0.8612, 5.9968) (0.7071, 6.2973) (0.6763, 7.0896) (0.822, 7.5702) knots 0 0 0 1 2 2 2
  spline S191 degree 2 poles (0.822, 7.5702) (0.9678, 8.0508) (1.4365, 8.6744) (1.7248, 8.8451) knots 0 0 0 1 2 2 2
  spline S192 degree 2 poles (1.7248, 8.8451) (2.0144, 9.0197) (2.7342, 9.0811) (3.1045, 8.9688) knots 0 0 0 1 2 2 2
  spline S193 degree 2 poles (3.1045, 8.9688) (3.4039, 8.878) (3.9119, 8.539) (4.0952, 8.363) knots 0 0 0 1 2 2 2
  line L165 (4.0952, 8.363) -> (3.8861, 7.6735)
  line L166 (3.8861, 7.6735) -> (3.8507, 7.6843)
  spline S194 degree 2 poles (3.8507, 7.6843) (3.8004, 7.7597) (3.6386, 7.9637) (3.5155, 8.0827) knots 0 0 0 1 2 2 2
  spline S195 degree 2 poles (3.5155, 8.0827) (3.4046, 8.1852) (3.0878, 8.3888) (2.9302, 8.4366) knots 0 0 0 1 2 2 2
  spline S196 degree 2 poles (2.9302, 8.4366) (2.4535, 8.5811) (1.6558, 8.0358) (1.4563, 7.3779) knots 0 0 0 1 2 2 2
  spline S197 degree 2 poles (1.4563, 7.3779) (1.2616, 6.7357) (1.6024, 5.8451) (2.0988, 5.6946) knots 0 0 0 1 2 2 2
  spline S198 degree 2 poles (2.0988, 5.6946) (2.3982, 5.6038) (3.0171, 5.6872) (3.2845, 5.8169) knots 0 0 0 1 2 2 2
  line L167 (3.2845, 5.8169) -> (3.3199, 5.8062)
  line L168 (3.3199, 5.8062) -> (3.1109, 5.1167)
  spline S199 degree 2 poles (3.1109, 5.1167) (3.0071, 5.1009) (2.6943, 5.0624) (2.5756, 5.0682) knots 0 0 0 1 2 2 2
  spline S200 degree 2 poles (2.5756, 5.0682) (2.4037, 5.0688) (2.1412, 5.0967) (1.9482, 5.1553) knots 0 0 0 1 2 2 2
  spline S201 degree 2 poles (4.461, 3.2273) (3.8881, 3.9393) (4.0571, 5.3645) (4.7948, 5.9581) knots 0 0 0 1 2 2 2
  spline S202 degree 2 poles (4.7948, 5.9581) (5.5197, 6.5413) (6.9909, 6.4727) (7.4838, 5.8601) knots 0 0 0 1 2 2 2
  spline S203 degree 2 poles (7.4838, 5.8601) (7.7057, 5.5843) (7.8886, 5.0286) (7.845, 4.7347) knots 0 0 0 1 2 2 2
  spline S204 degree 2 poles (7.845, 4.7347) (7.804, 4.4376) (7.4501, 3.8727) (7.0941, 3.5863) knots 0 0 0 1 2 2 2
  line L169 (7.0941, 3.5863) -> (6.8214, 3.3669)
  line L170 (6.8214, 3.3669) -> (5.1673, 5.4229)
  spline S205 degree 2 poles (5.1673, 5.4229) (4.6509, 5.0074) (4.5204, 4.0465) (4.8921, 3.5847) knots 0 0 0 1 2 2 2
  spline S206 degree 2 poles (4.8921, 3.5847) (5.0237, 3.4211) (5.3529, 3.1629) (5.5139, 3.081) knots 0 0 0 1 2 2 2
  spline S207 degree 2 poles (5.5139, 3.081) (5.6864, 2.9979) (5.9483, 2.9022) (6.0487, 2.8826) knots 0 0 0 1 2 2 2
  line L171 (6.0487, 2.8826) -> (6.0719, 2.8537)
  line L172 (6.0719, 2.8537) -> (5.5267, 2.415)
  spline S208 degree 2 poles (5.5267, 2.415) (5.4217, 2.4732) (5.1075, 2.6537) (4.996, 2.7331) knots 0 0 0 1 2 2 2
  spline S209 degree 2 poles (4.996, 2.7331) (4.8382, 2.8439) (4.6055, 3.0477) (4.461, 3.2273) knots 0 0 0 1 2 2 2
  spline S210 degree 2 poles (6.8109, 4.1616) (7.0078, 4.3305) (7.2358, 4.6514) (7.2707, 4.8115) knots 0 0 0 1 2 2 2
  spline S211 degree 2 poles (7.2707, 4.8115) (7.3133, 4.9885) (7.2126, 5.3566) (7.05, 5.5586) knots 0 0 0 1 2 2 2
  spline S212 degree 2 poles (7.05, 5.5586) (6.89, 5.7575) (6.5468, 5.9411) (6.3384, 5.9636) knots 0 0 0 1 2 2 2
  spline S213 degree 2 poles (6.3384, 5.9636) (6.1294, 5.9804) (5.7511, 5.8662) (5.5489, 5.73) knots 0 0 0 1 2 2 2
  line L173 (5.5489, 5.73) -> (6.8109, 4.1616)
  spline S214 degree 2 poles (6.5024, -4.2871) (5.6082, -3.9515) (4.8719, -2.7034) (5.1163, -2.052) knots 0 0 0 1 2 2 2
  spline S215 degree 2 poles (5.1163, -2.052) (5.2161, -1.7861) (5.4928, -1.4238) (5.6995, -1.2596) knots 0 0 0 1 2 2 2
  line L174 (5.6995, -1.2596) -> (4.2041, -0.6984)
  line L175 (4.2041, -0.6984) -> (4.4297, -0.0971)
  line L176 (4.4297, -0.0971) -> (9.313, -1.9298)
  line L177 (9.313, -1.9298) -> (9.0874, -2.531)
  line L178 (9.0874, -2.531) -> (8.7135, -2.3907)
  spline S216 degree 2 poles (8.7135, -2.3907) (8.8339, -2.6909) (8.8983, -3.3395) (8.7782, -3.6594) knots 0 0 0 1 2 2 2
  spline S217 degree 2 poles (8.7782, -3.6594) (8.5482, -4.2722) (7.3195, -4.5937) (6.5024, -4.2871) knots 0 0 0 1 2 2 2
  spline S218 degree 2 poles (6.6659, -3.6405) (7.2787, -3.8705) (8.0993, -3.7344) (8.2628, -3.2989) knots 0 0 0 1 2 2 2
  spline S219 degree 2 poles (8.2628, -3.2989) (8.3582, -3.0445) (8.3102, -2.4812) (8.2125, -2.2027) knots 0 0 0 1 2 2 2
  line L179 (8.2125, -2.2027) -> (6.1852, -1.4419)
  spline S220 degree 2 poles (6.1852, -1.4419) (5.9852, -1.635) (5.7745, -1.9385) (5.6935, -2.1543) knots 0 0 0 1 2 2 2
  spline S221 degree 2 poles (5.6935, -2.1543) (5.5185, -2.6207) (6.0107, -3.3946) (6.6659, -3.6405) knots 0 0 0 1 2 2 2
  line L180 (3.6863, -8.8133) -> (2.8107, -4.8347)
  line L181 (2.8107, -4.8347) -> (3.2937, -4.5203)
  line L182 (3.2937, -4.5203) -> (6.5671, -6.938)
  line L183 (6.5671, -6.938) -> (5.984, -7.3175)
  line L184 (5.984, -7.3175) -> (3.5099, -5.4258)
  line L185 (3.5099, -5.4258) -> (4.2452, -8.4495)
  line L186 (4.2452, -8.4495) -> (3.6863, -8.8133)
  spline S222 degree 2 poles (-2.06, -8.0262) (-1.9866, -6.6614) (-1.1245, -5.4256) (-0.2982, -5.4701) knots 0 0 0 1 2 2 2
  spline S223 degree 2 poles (-0.2982, -5.4701) (0.5403, -5.5151) (1.2554, -6.8605) (1.1836, -8.1965) knots 0 0 0 1 2 2 2
  spline S224 degree 2 poles (1.1836, -8.1965) (1.1098, -9.5695) (0.2481, -10.797) (-0.5823, -10.7524) knots 0 0 0 1 2 2 2
  spline S225 degree 2 poles (-0.5823, -10.7524) (-1.4168, -10.7075) (-2.1312, -9.3498) (-2.06, -8.0262) knots 0 0 0 1 2 2 2
  spline S226 degree 2 poles (-1.1054, -6.5274) (-1.2176, -6.7728) (-1.3413, -7.5413) (-1.3694, -8.0633) knots 0 0 0 1 2 2 2
  spline S227 degree 2 poles (-1.3694, -8.0633) (-1.3975, -8.5854) (-1.3566, -9.3585) (-1.2677, -9.623) knots 0 0 0 1 2 2 2
  spline S228 degree 2 poles (-1.2677, -9.623) (-1.1789, -9.8875) (-0.8356, -10.174) (-0.552, -10.1892) knots 0 0 0 1 2 2 2
  spline S229 degree 2 poles (-0.552, -10.1892) (-0.2684, -10.2045) (0.1119, -9.9569) (0.2331, -9.6955) knots 0 0 0 1 2 2 2
  spline S230 degree 2 poles (0.2331, -9.6955) (0.3498, -9.442) (0.4662, -8.6567) (0.493, -8.1593) knots 0 0 0 1 2 2 2
  spline S231 degree 2 poles (0.493, -8.1593) (0.5217, -7.6249) (0.4944, -6.9061) (0.4026, -6.6208) knots 0 0 0 1 2 2 2
  spline S232 degree 2 poles (0.4026, -6.6208) (0.3181, -6.3525) (-0.0326, -6.0491) (-0.3285, -6.0332) knots 0 0 0 1 2 2 2
  spline S233 degree 2 poles (-0.3285, -6.0332) (-0.6081, -6.0182) (-0.9883, -6.2657) (-1.1054, -6.5274) knots 0 0 0 1 2 2 2
  line L187 (-6.0992, -4.4207) -> (-5.6408, -4.8158)
  line L188 (-5.6408, -4.8158) -> (-4.5011, -3.4938)
  line L189 (-4.5011, -3.4938) -> (-4.0054, -3.9212)
  line L190 (-4.0054, -3.9212) -> (-5.1451, -5.2432)
  line L191 (-5.1451, -5.2432) -> (-3.4458, -6.7082)
  line L192 (-3.4458, -6.7082) -> (-3.9135, -7.2507)
  line L193 (-3.9135, -7.2507) -> (-7.3441, -7.75)
  line L194 (-7.3441, -7.75) -> (-7.8181, -7.3414)
  line L195 (-7.8181, -7.3414) -> (-5.9983, -5.2305)
  line L196 (-5.9983, -5.2305) -> (-6.4567, -4.8354)
  line L197 (-6.4567, -4.8354) -> (-6.0992, -4.4207)
  line L198 (-5.5026, -5.6579) -> (-6.7982, -7.1608)
  line L199 (-6.7982, -7.1608) -> (-4.2086, -6.7734)
  line L200 (-4.2086, -6.7734) -> (-5.5026, -5.6579)
  dimension "d9" = 33.02
  constraints: 1 centre point, 1 coincident, 1 other
  measures "d9" diameter of A0
emboss "Emboss1" sketch "Sketch4" operation cut depth 1.27 direction (0, 0, 1)
sketch "Sketch6" plane through (-3.6662, 6.35, 17.4625) normal (0, 1, 0) x (1, 0, 0)
  line L0 (7.3323, 0) -> (0, 0) construction
  line L1 (3.6662, 0) -> (3.6662, 34.6111) construction
  line L2 (19.4142, 34.925) -> (-12.0818, 34.925) projected
  point P0 (3.6662, 17.4625)
  point P1 (3.6662, 4.511)
  point P2 (3.6662, 28.7274)
  dimension "d12" = 4.511
  dimension "d13" = 6.1976
  constraints: 2 end point, 2 point on line, 1 midpoint, 1 vertical
  measures "d12" distance from line of point (3.666, 4.511) L0
  measures "d13" distance from line of point (3.666, 28.727) L2
hole "Hole1" at (0, 6.35, 12.9515) at (0, 6.35, -11.2649) direction (0, -1, 0) diameter 4.318 end through all clearance for "Hex Machine Screw" size "#6" standard "Ansi Unified Screw Threads"
equation "\"d0\" = printedHexSize"
equation "\"d1\" = length"
equation "\"hexSize\" = 12.7"
equation "\"slipFitOffset\" = 0"
equation "\"printedHexSize\" = hexSize - slipFitOffset"
equation "\"length\" = 34.925"
equation "\"bushingSlipOffset\" = 0.381"
body "Solid1"
